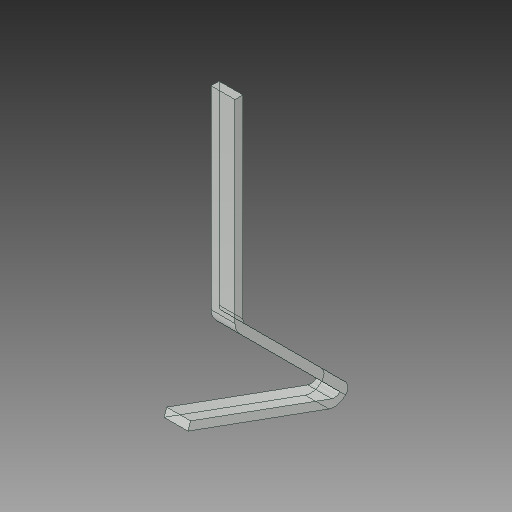
# Autodesk Inventor part: Plexi hooks
Saved by Autodesk Inventor 2019 (Build 230136000, 136)
## iProperties
Created: 2019-02-27
Part Number: Plexi hooks
Material: Generic
Document SubType Name: Modeling
Designer: josh
Density: 1 g/cm^3
Appearance: Clear
Mass: 49.7337 g
Surface Area: 211.275 cm^2
Volume: 49.7337 cm^3
Author: josh
Autodesk Inventor part; units mm, degrees
note: some values were not read from the file. Chosen so that the rebuilt part matches the saved one: bend side of "Bend Part2".
ref_plane "YZ Plane" through (0, 0, 0) normal (1, 0, 0) x (0, 1, 0)
ref_plane "XZ Plane" through (0, 0, 0) normal (0, 1, 0) x (-1, 0, 0)
ref_plane "XY Plane" through (0, 0, 0) normal (0, 0, 1) x (1, 0, 0)
sketch "Sketch1" plane through (0, 0, 0) normal (1, 0, 0) x (0, 1, 0)
  line L0 (6.35, -12.9887) -> (279.4, -12.9887)
  line L1 (279.4, -12.9887) -> (279.4, -19.3387)
  line L2 (279.4, -19.3387) -> (0, -19.3387)
  line L3 (0, -19.3387) -> (0, -12.9887)
  line L4 (0, -12.9887) -> (0, 114.0113)
  line L5 (0, 114.0113) -> (6.35, 114.0113)
  line L6 (6.35, 114.0113) -> (6.35, -12.9887)
  point P0 (0, 0)
  dimension "d0" = 279.4
  dimension "d1" = 6.35
  dimension "d2" = 127
  dimension "d3" = 6.35
  constraints: 14 end point, 4 perpendicular, 1 horizontal, 1 parallel, 1 point on line
  measures "d0" distance of L3.end L0.end
  measures "d1" distance of L0.end L1.end
  measures "d2" distance of L3.end L4.end
  measures "d3" distance of L4.end L5.end
extrude "Extrusion1" add sketch "Sketch1" against normal blind 19.05
sketch "Sketch2" plane through (0, 6.35, 114.0113) normal (0, 1, 0) x (1, 0, 0)
  line L0 (0, 127) -> (-19.05, 127) projected
  line L1 (-19.05, 127) -> (0, 127)
  line L2 (0, 0) -> (0, 133.35) projected
  point P0 (0, 114.0113)
  constraints: 2 end point, 1 perpendicular
fillet "Fillet1" radius 6.35 1 edges at (-9.525, 0, -19.3387)
bend part "Bend Part1" radius 6.35 angle 65 line through (-19.05, 6.35, -12.9887) along (1, 0, 0) centre toward (0, 1, 0) moving side (0, 0, 1) both sides no
sketch "Sketch3" plane through (0, 6.35, -19.3387) normal (0, 0, -1) x (-1, 0, 0)
  line L0 (39.6982, 130.9983) -> (-135.4768, 130.9983) projected
  line L1 (19.05, 118.2983) -> (0, 118.2983)
  point P0 (0, -6.35)
  constraints: 2 end point
bend part "Bend Part2" radius 6.35 angle 45 line through (-19.05, 124.6483, -19.3387) along (1, 0, 0) centre toward (0, 0, -1) moving side (0, -1, 0) both sides no
body "Solid1"
